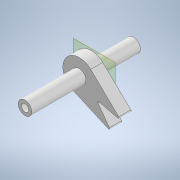
# Autodesk Inventor part: reverser-base
Saved by Autodesk Inventor 2022 (Build 260153000, 153)
## iProperties
Created: 2021-07-09
Part Number: reverser-base
Material: Generic
Document SubType Name: Modeling
Designer: teh18
Density: 1 g/cm^3
Appearance: Default
Mass: 12.077 g
Surface Area: 54.5901 cm^2
Volume: 12.077 cm^3
Author: teh18
Autodesk Inventor part; units mm, degrees
ref_plane "YZ Plane" through (0, 0, 0) normal (1, 0, 0) x (0, 1, 0)
ref_plane "XZ Plane" through (0, 0, 0) normal (0, 1, 0) x (-1, 0, 0)
ref_plane "XY Plane" through (0, 0, 0) normal (0, 0, 1) x (1, 0, 0)
sketch "Sketch1" plane through (0, 0, 0) normal (0, 0, 1) x (1, 0, 0)
  line L0 (2.6, -0.6) -> (-2.6, -0.6) projected
  line L1 (-2.6, -0.6) -> (-2.6, 0.6) projected
  line L2 (-2.6, 0.6) -> (2.6, 0.6) projected
  line L3 (2.6, 0.6) -> (2.6, -0.6) projected
  circle A0 centre (0, 0) radius 3.6 projected
  line L4 (-2.7, 0.7) -> (-2.7, -0.7)
  line L5 (-2.7, -0.7) -> (2.7, -0.7)
  line L6 (2.7, -0.7) -> (2.7, 0.7)
  line L7 (2.7, 0.7) -> (-2.7, 0.7)
  circle A1 centre (0, 0) radius 5.6
  dimension "d0" = 0.1
  dimension "d5" = 2
  constraints: 8 end point, 1 centre point, 3 other
  measures "d0" distance between parallel lines of L1 L4
  measures "d5" radial gap between concentric circles of A0 A1
extrude "Extrusion1" add sketch "Sketch1" along normal blind 10 contours A0 | A1
sketch "Sketch2" plane through (0, 0, 10) normal (0, 0, 1) x (0, -1, 0)
  line L0 (-0.7, -2.7) -> (-0.7, 2.7) projected
  line L1 (-0.7, 2.7) -> (0.7, 2.7) projected
  line L2 (0.7, 2.7) -> (0.7, -2.7) projected
  line L3 (0.7, -2.7) -> (-0.7, -2.7) projected
  circle A0 centre (0, 0) radius 3.75
  circle A1 centre (0, 0) radius 5.6 projected
  constraints: 1 centre point, 2 other
ref_plane "Work Plane1" through (-14, -11, 93) normal (0, 0, -1) x (0, 1, 0)
extrude "Extrusion2" add sketch "Sketch2" along normal blind 80 contours L0 L1 L2 L3 | A0 | A1
ref_plane "Work Plane2" through (14.5169, -8.0562, 35) normal (0, 0, -1) x (-1, 0, 0)
sketch "Sketch4" plane through (0, 0, 90) normal (0, 0, 1) x (1, 0, 0)
  circle A0 centre (0, 0) radius 3
  dimension "d20" = 6
  constraints: 1 centre point, 1 coincident
  measures "d20" diameter of A0
extrude "Extrusion4" cut sketch "Sketch4" against normal blind 10
sketch "Sketch5" plane through (0, 0, 80) normal (0, 0, 1) x (1, 0, 0)
  circle A0 centre (0, 0) radius 3 projected
  circle A1 centre (0, 0) radius 3 projected
  line L0 (-3, 0.5) -> (3, 0.5)
  line L1 (3, 0.5) -> (3, -0.5)
  line L2 (3, -0.5) -> (-3, -0.5)
  line L3 (-3, -0.5) -> (-3, 0.5)
  line L4 (-3, 0.5) -> (3, -0.5) construction
  line L5 (3, 0.5) -> (-3, -0.5) construction
  point P0 (-2.958, -0.5)
  point P1 (2.958, -0.5)
  point P2 (2.958, 0.5)
  point P3 (-2.958, 0.5)
  dimension "d24" = 6
  dimension "d25" = 1
  constraints: 12 end point, 2 midpoint, 2 parallel, 1 horizontal, 1 perpendicular
  measures "d24" distance of L1.end L2.end
  measures "d25" distance of L0.end L1.end
extrude "Extrusion5" add sketch "Sketch5" along normal blind 0.8 contours A0 L2 L0
sketch "Sketch6" plane through (14.5169, -8.0562, 35) normal (0, 0, -1) x (-1, 0, 0)
  circle A0 centre (14.5169, 8.0562) radius 5.6 projected
  circle A1 centre (14.5169, 8.0562) radius 13.6
  line L0 (19.2509, -4.6933) -> (-8.8851, -15.1405)
  line L1 (4.1919, 16.9079) -> (-15.3464, -5.8823)
  line L2 (-8.8851, -15.1405) -> (0.2779, -1.8727)
  line L3 (0.2779, -1.8727) -> (-15.3464, -5.8823)
  line L4 (20.3441, -4.2322) -> (-52.8556, -38.9438)
  line L5 (4.1919, 16.9079) -> (-52.8556, -38.9438)
  arc A2 (-101.4982, -27.3726) -> (-98.3101, -29.4028) centre (-99.5525, -27.8355) ccw
  arc A3 (-98.7514, -19.105) -> (-101.4982, -27.3726) centre (-52.8556, -38.9438) ccw
  line L6 (-98.7514, -19.105) -> (-109.7663, -14.3437)
  arc A4 (-98.2472, 3.2889) -> (-109.7663, -14.3437) centre (-52.8556, -38.9438) ccw
  line L7 (-98.2472, 3.2889) -> (-89.4617, -4.8852)
  arc A5 (-18.7969, -2.3377) -> (-89.4617, -4.8852) centre (-52.8556, -38.9438) ccw
  line L8 (-18.7969, -2.3377) -> (-26.971, -11.1232)
  arc A6 (-41.1368, -75.0917) -> (-26.971, -11.1232) centre (-52.8556, -38.9438) ccw
  line L9 (-41.1368, -75.0917) -> (-42.3055, -71.487)
  arc A7 (-42.3055, -71.487) -> (-59.8761, -67.1138) centre (-52.9931, -76.9436) ccw
  arc A8 (-61.0624, -66.7913) -> (-59.8761, -67.1138) centre (-60.3349, -66.4585) ccw
  arc A9 (-61.0624, -66.7913) -> (-73.0205, -59.8295) centre (-71.9745, -71.7838) ccw
  arc A10 (-73.8866, -58.957) -> (-73.0205, -59.8295) centre (-73.0902, -59.0325) ccw
  arc A11 (-73.8866, -58.957) -> (-80.7617, -46.9489) centre (-85.8331, -57.8246) ccw
  arc A12 (-81.0756, -45.7602) -> (-80.7617, -46.9489) centre (-80.4236, -46.2238) ccw
  arc A13 (-81.0756, -45.7602) -> (-85.3215, -28.1585) centre (-90.8553, -38.8063) ccw
  line L10 (-85.3215, -28.1585) -> (-88.9177, -26.9638)
  arc A14 (-88.9177, -26.9638) -> (-98.3101, -29.4028) centre (-90.8553, -38.8063) ccw
  circle A15 centre (-52.8556, -38.9438) radius 4
  circle A16 centre (-52.8556, -38.9438) radius 18
  circle A17 centre (-52.8556, -38.9438) radius 50
  line L11 (0.2779, -1.8727) -> (-52.8556, -38.9438)
  point P0 (2.5698, 1.558)
  point P1 (4.2932, -0.9124)
  dimension "d30" = 8
  dimension "d34" = 35
  dimension "d36" = 5
  dimension "d37" = 5
  dimension "d39" = 35
  constraints: 32 point on circle, 24 end point, 17 centre point, 3 tangent, 2 coincident, 1 line through centre, 54 other
  measures "d30" radial gap between concentric circles of A0 A1
  measures "d34" angle of L2 L0
  measures "d36" angle of L0 L4
  measures "d37" angle of L5 L1
  measures "d39" angle of L1 L3
extrude "Extrusion6" add sketch "Sketch6" against normal blind 10 contours A1 | A1 L0 L2 L3 L1
fillet "Fillet1" radius 2.5 3 edges at (23.402, -23.1967, 40) (29.8633, -13.9385, 40) (14.2391, -9.9288, 40)
equation "\"d37\" = d36"
equation "\"d39\" = d34"
body "Solid1"
